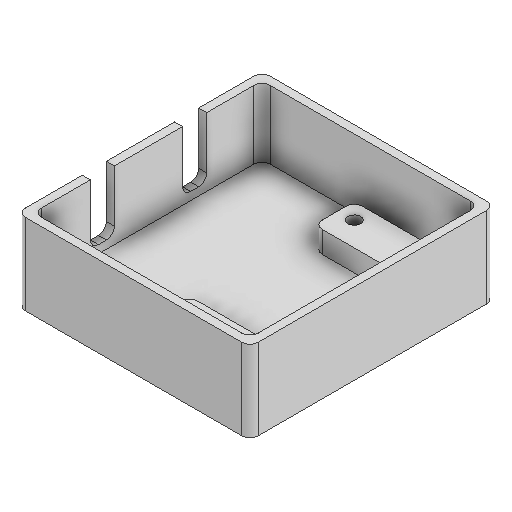
# Autodesk Inventor part: 3DP_ASA_Preamp_Case_Top
Saved by Autodesk Inventor 2026.1 (Build 301233000, 233)
## iProperties
Created: 2025-06-27
Part Number: 3DP_ASA_Preamp_Case_Top
Material: Generic
Document SubType Name: Modeling
Designer: User
Density: 1 g/cm^3
Appearance: Default
Author: User
Autodesk Inventor part; units mm, degrees
ref_plane "YZ Plane" through (0, 0, 0) normal (1, 0, 0) x (0, 1, 0)
ref_plane "XZ Plane" through (0, 0, 0) normal (0, 1, 0) x (-1, 0, 0)
ref_plane "XY Plane" through (0, 0, 0) normal (0, 0, 1) x (1, 0, 0)
sketch "Sketch1" plane through (0, 0, 0) normal (0, 1, 0) x (-1, 0, 0)
  line L0 (12.5, 25.5) -> (-12.5, 25.5)
  line L1 (-12.5, 25.5) -> (-12.5, -25.5)
  line L2 (-12.5, -25.5) -> (12.5, -25.5)
  line L3 (12.5, -25.5) -> (12.5, 25.5)
  line L4 (13, 26) -> (-13, 26)
  line L5 (-13, 26) -> (-13, -26)
  line L6 (-13, -26) -> (13, -26)
  line L7 (13, -26) -> (13, 26)
  line L8 (15, 28) -> (-15, 28)
  line L9 (-15, 28) -> (-15, -28)
  line L10 (-15, -28) -> (15, -28)
  circle A0 centre (8.5, 21.5) radius 1.6
  circle A1 centre (8.5, -21.5) radius 1.6
  circle A2 centre (-8.5, 21.5) radius 1.6
  circle A3 centre (-8.5, -21.5) radius 1.6
  line L11 (15, -28) -> (38, -28)
  line L12 (38, -28) -> (38, -26)
  line L13 (38, -26) -> (13, -26)
  line L14 (13, 26) -> (38, 26)
  line L15 (38, 26) -> (38, 28)
  line L16 (38, 28) -> (15, 28)
  line L17 (38, -26) -> (38, 26)
  line L18 (12.5, -15.5) -> (-12.5, -15.5)
  line L19 (12.5, 15.5) -> (-12.5, 15.5)
  line L20 (12.5, -15.5) -> (13, -15.5)
  line L21 (12.5, 15.5) -> (13, 15.5)
  line L22 (-12.5, -15.5) -> (-13, -15.5)
  line L23 (-12.5, 15.5) -> (-13, 15.5)
  line L24 (38.5, -26) -> (38.5, -28.5)
  line L25 (38.5, -28.5) -> (15, -28.5)
  line L26 (15, -28.5) -> (-15.5, -28.5)
  line L27 (-15.5, -28.5) -> (-15.5, 28.5)
  line L28 (-15.5, 28.5) -> (15, 28.5)
  line L29 (15, 28.5) -> (38.5, 28.5)
  line L30 (38.5, 28.5) -> (38.5, 26)
  line L31 (38.5, -26) -> (38, -26)
  line L32 (38.5, 26) -> (38, 26)
  line L33 (38, 24) -> (40.5, 24)
  line L34 (40.5, 24) -> (40.5, 30.5)
  line L35 (40.5, 30.5) -> (-17.5, 30.5)
  line L36 (-17.5, 30.5) -> (-17.5, -30.5)
  line L37 (-17.5, -30.5) -> (15, -30.5)
  line L38 (15, -30.5) -> (40.5, -30.5)
  line L39 (40.5, -30.5) -> (40.5, -24)
  line L40 (40.5, -24) -> (38, -24)
  line L41 (40.5, -24) -> (40.5, 24)
  line L42 (38.5, -26) -> (38.5, -24)
  line L43 (38.5, -24) -> (38.5, 24)
  line L44 (38.5, 24) -> (38.5, 26)
  point P0 (0, 0)
  dimension "d0" = 51
  dimension "d1" = 25
  dimension "d2" = 12.5
  dimension "d3" = 25.5
  dimension "d4" = 4
  dimension "d5" = 4
  dimension "d6" = 4
  dimension "d7" = 4
  dimension "d8" = 0.5
  dimension "d10" = 3.2
  dimension "d11" = 3.2
  dimension "d12" = 3.2
  dimension "d13" = 3.2
  dimension "d50" = 25
  dimension "d51" = 10
  dimension "d52" = 10
  dimension "d69" = 0.5
  dimension "d70" = 2
  constraints: 90 end point, 18 perpendicular, 11 point on line, 9 parallel, 4 centre point, 4 coincident, 4 horizontal, 2 horizontal alignment, 2 vertical, 2 vertical alignment, 1 collinear, 18 other
  measures "d0" distance between parallel lines of L2 L0
  measures "d1" distance of L1.end L2.end
  measures "d2" distance from line of L3 point (0, 0)
  measures "d3" distance from line of L2 point (0, 0)
  measures "d4" distance from line of L0 point (8.5, 21.5)
  measures "d5" distance from line of L3 point (8.5, 21.5)
  measures "d6" distance from line of L1 point (-8.5, 21.5)
  measures "d7" distance from line of L2 point (8.5, -21.5)
  measures "d8" distance between parallel lines of L3 L7
  measures "d10" diameter of A0
  measures "d11" diameter of A1
  measures "d12" diameter of A2
  measures "d13" diameter of A3
  measures "d50" distance between parallel lines of L17 L7
  measures "d51" distance between parallel lines of L2 L18
  measures "d52" distance between parallel lines of L0 L19
  measures "d69" distance between parallel lines of L11 L25
  measures "d70" distance between parallel lines of L27 L36
extrude "Extrusion1" add sketch "Sketch1" against normal blind 3.2
extrude "Extrusion2" add sketch "Sketch1" along normal blind 17 contours L30 L29 L28 L27 L26 L25 L24 L42 L40 L39 L38 L37 L36 L35 L34 L33 L44 | L33 L41 L40 L43
extrude "Extrusion11" add sketch "Sketch1" along normal blind 5.4 contours L3 L19 L1 L0 | L3 L2 L1 L18
fillet "Fillet6" radius 2 8 edges at (-40.5, 6.9, 30.5) (-40.5, 6.9, -30.5) (17.5, 6.9, -30.5) (17.5, 6.9, 30.5) (15.5, 8.5, 28.5) (15.5, 8.5, -28.5) (-38.5, 8.5, -28.5) (-38.5, 8.5, 28.5)
fillet "Fillet7" radius 2 8 edges at (-12.5, 2.7, -15.5) (-12.5, 2.7, -25.5) (12.5, 2.7, -15.5) (12.5, 2.7, -25.5) (12.5, 2.7, 15.5) (12.5, 2.7, 25.5) (-12.5, 2.7, 25.5) (-12.5, 2.7, 15.5)
sketch "Sketch9" plane through (-40.5, -3.2, -28.5) normal (-1, 0, 0) x (0, 0, 1)
  line L0 (59, 0) -> (59, 20.2) projected
  line L1 (0, 0) -> (0, 20.2) projected
  line L2 (57, 0) -> (0, 0) projected
  line L3 (57, 20.2) -> (57, 0) projected
  line L4 (0, 20.2) -> (57, 20.2) projected
  line L5 (57, 20.2) -> (59, 20.2) projected
  line L6 (59, 0) -> (57, 0) projected
  line L7 (-2, 20.2) -> (0, 20.2) projected
  line L8 (0, 0) -> (-2, 0) projected
  line L9 (-2, 20.2) -> (-2, 0) projected
  line L10 (42.8, 20.2) -> (42.8, 5.2)
  line L11 (42.8, 5.2) -> (36.8, 5.2)
  line L12 (36.8, 5.2) -> (36.8, 20.2)
  line L13 (19.8, 20.2) -> (19.8, 5.2)
  line L14 (19.8, 5.2) -> (13.8, 5.2)
  line L15 (13.8, 5.2) -> (13.8, 20.2)
  point P0 (28.5, 3.2)
  dimension "d75" = 6
  dimension "d76" = 15
  dimension "d77" = 6
  dimension "d78" = 16.2
  dimension "d79" = 17
  constraints: 12 end point, 6 point on line, 3 perpendicular, 1 parallel, 1 vertical
  measures "d75" distance between parallel lines of L12 L10
  measures "d76" distance between parallel lines of L4 L11
  measures "d77" distance between parallel lines of L15 L13
  measures "d78" distance between parallel lines of L10 L0
  measures "d79" distance between parallel lines of L13 L12
extrude "Extrusion12" cut sketch "Sketch9" against normal blind 5.4 contours L10 L11 L12 L4 | L4 L13 L14 L15
fillet "Fillet8" radius 2 4 edges at (-39.5, 2, 14.3) (-39.5, 2, 8.3) (-39.5, 2, -8.7) (-39.5, 2, -14.7)
sketch "Sketch10" plane through (0, -3.2, 0) normal (0, -1, 0) x (1, 0, 0)
  line L0 (-23.4723, 25.4244) -> (-23.4723, -0.8586) construction
  line L1 (-23.4723, -0.8586) -> (-26.6245, -0.8586) construction
  line L2 (-26.6245, -0.8586) -> (-26.6245, 25.4244) construction
  line L3 (-26.6245, 25.4244) -> (-23.4723, 25.4244) construction
  line L4 (-23.5729, 24.8116) -> (-23.5729, 22.4106)
  spline S0 degree 2 poles (-23.5729, 22.4106) (-23.5729, 21.6972) (-23.6918, 20.9975) (-24.0668, 20.4442) (-24.6933, 20.0738) (-25.082, 20.0738) knots 0 0 0 1 2 3 4 4 4
  spline S1 degree 2 poles (-25.082, 20.0738) (-25.5027, 20.0738) (-26.2024, 20.5265) (-26.3808, 20.9152) knots 0 0 0 1 2 2 2
  spline S2 degree 2 poles (-26.3808, 20.9152) (-26.5409, 20.3664) (-27.3091, 19.7811) (-27.8305, 19.7811) knots 0 0 0 1 2 2 2
  spline S3 degree 2 poles (-27.8305, 19.7811) (-28.2421, 19.7811) (-29.0149, 20.1606) (-29.4768, 20.8238) (-29.5317, 21.3039) knots 0 0 0 1 2 3 3 3
  spline S4 degree 2 poles (-29.5317, 21.3039) (-29.5637, 21.6103) (-29.5729, 22.7674) knots 0 0 0 1 1 1
  line L5 (-29.5729, 22.7674) -> (-29.5729, 24.8116)
  line L6 (-29.5729, 24.8116) -> (-23.5729, 24.8116)
  line L7 (-26.9524, 23.5997) -> (-28.5576, 23.5997)
  line L8 (-28.5576, 23.5997) -> (-28.5576, 22.4747)
  spline S5 degree 2 poles (-28.5576, 22.4747) (-28.5576, 21.8161) (-28.521, 21.6424) knots 0 0 0 1 1 1
  spline S6 degree 2 poles (-28.521, 21.6424) (-28.4707, 21.3725) (-28.0912, 21.0295) (-27.771, 21.0295) knots 0 0 0 1 2 2 2
  spline S7 degree 2 poles (-27.771, 21.0295) (-27.5012, 21.0295) (-27.1262, 21.2902) (-26.9524, 21.7887) (-26.9524, 22.6164) knots 0 0 0 1 2 3 3 3
  line L9 (-26.9524, 22.6164) -> (-26.9524, 23.5997)
  line L10 (-24.5698, 23.5997) -> (-25.9555, 23.5997)
  line L11 (-25.9555, 23.5997) -> (-25.9555, 22.8039)
  spline S8 degree 2 poles (-25.9555, 22.8039) (-25.9555, 22.0951) (-25.9372, 21.9213) knots 0 0 0 1 1 1
  spline S9 degree 2 poles (-25.9372, 21.9213) (-25.896, 21.6103) (-25.5439, 21.2536) (-25.2512, 21.2536) knots 0 0 0 1 2 2 2
  spline S10 degree 2 poles (-25.2512, 21.2536) (-24.9723, 21.2536) (-24.6293, 21.56) (-24.5881, 21.8664) knots 0 0 0 1 2 2 2
  spline S11 degree 2 poles (-24.5881, 21.8664) (-24.5698, 22.0448) (-24.5698, 22.9045) knots 0 0 0 1 1 1
  line L12 (-24.5698, 22.9045) -> (-24.5698, 23.5997)
  line L13 (-29.5729, 17.1835) -> (-27.0485, 17.1835)
  line L14 (-27.0485, 17.1835) -> (-23.5729, 19.3786)
  line L15 (-23.5729, 19.3786) -> (-23.5729, 17.9609)
  line L16 (-23.5729, 17.9609) -> (-25.9509, 16.5433)
  line L17 (-25.9509, 16.5433) -> (-23.5729, 15.1622)
  line L18 (-23.5729, 15.1622) -> (-23.5729, 13.7628)
  line L19 (-23.5729, 13.7628) -> (-27.0576, 15.9716)
  line L20 (-27.0576, 15.9716) -> (-29.5729, 15.9716)
  line L21 (-29.5729, 15.9716) -> (-29.5729, 17.1835)
  line L22 (-29.5729, 11.8146) -> (-24.5881, 11.8146)
  line L23 (-24.5881, 11.8146) -> (-24.5881, 13.5936)
  line L24 (-24.5881, 13.5936) -> (-23.5729, 13.5936)
  line L25 (-23.5729, 13.5936) -> (-23.5729, 8.8283)
  line L26 (-23.5729, 8.8283) -> (-24.5881, 8.8283)
  line L27 (-24.5881, 8.8283) -> (-24.5881, 10.6027)
  line L28 (-24.5881, 10.6027) -> (-29.5729, 10.6027)
  line L29 (-29.5729, 10.6027) -> (-29.5729, 11.8146)
  line L30 (-29.5729, 8.0417) -> (-23.5729, 8.0417)
  line L31 (-23.5729, 8.0417) -> (-23.5729, 3.592)
  line L32 (-23.5729, 3.592) -> (-24.5881, 3.592)
  line L33 (-24.5881, 3.592) -> (-24.5881, 6.8299)
  line L34 (-24.5881, 6.8299) -> (-25.9189, 6.8299)
  line L35 (-25.9189, 6.8299) -> (-25.9189, 3.8161)
  line L36 (-25.9189, 3.8161) -> (-26.9341, 3.8161)
  line L37 (-26.9341, 3.8161) -> (-26.9341, 6.8299)
  line L38 (-26.9341, 6.8299) -> (-28.5576, 6.8299)
  line L39 (-28.5576, 6.8299) -> (-28.5576, 3.4777)
  line L40 (-28.5576, 3.4777) -> (-29.5729, 3.4777)
  line L41 (-29.5729, 3.4777) -> (-29.5729, 8.0417)
  line L42 (-27.364, -1.3881) -> (-27.7345, -2.5634)
  spline S12 degree 2 poles (-27.7345, -2.5634) (-28.7177, -2.2936) (-29.6735, -1.036) (-29.6735, -0.0711) knots 0 0 0 1 2 2 2
  spline S13 degree 2 poles (-29.6735, -0.0711) (-29.6735, 1.1225) (-28.0409, 2.6637) (-26.6277, 2.6637) knots 0 0 0 1 2 2 2
  spline S14 degree 2 poles (-26.6277, 2.6637) (-25.1277, 2.6637) (-23.4723, 1.118) (-23.4723, -0.1442) knots 0 0 0 1 2 2 2
  spline S15 degree 2 poles (-23.4723, -0.1442) (-23.4723, -1.2418) (-24.1216, -1.9323) knots 0 0 0 1 1 1
  spline S16 degree 2 poles (-24.1216, -1.9323) (-24.5058, -2.3394) (-25.2238, -2.5451) knots 0 0 0 1 1 1
  line L43 (-25.2238, -2.5451) -> (-25.5119, -1.347)
  spline S17 degree 2 poles (-25.5119, -1.347) (-25.0454, -1.2418) (-24.5058, -0.565) (-24.5058, -0.0848) knots 0 0 0 1 2 2 2
  spline S18 degree 2 poles (-24.5058, -0.0848) (-24.5058, 0.5829) (-25.4616, 1.4152) (-26.5363, 1.4152) knots 0 0 0 1 2 2 2
  spline S19 degree 2 poles (-26.5363, 1.4152) (-27.675, 1.4152) (-28.6399, 0.5966) (-28.6399, -0.0573) knots 0 0 0 1 2 2 2
  spline S20 degree 2 poles (-28.6399, -0.0573) (-28.6399, -0.5421) (-28.0226, -1.2372) (-27.364, -1.3881) knots 0 0 0 1 2 2 2
  line L44 (-29.5729, -3.6061) -> (-23.5729, -3.6061)
  line L45 (-23.5729, -3.6061) -> (-23.5729, -4.818)
  line L46 (-23.5729, -4.818) -> (-25.9326, -4.818)
  line L47 (-25.9326, -4.818) -> (-25.9326, -7.1915)
  line L48 (-25.9326, -7.1915) -> (-23.5729, -7.1915)
  line L49 (-23.5729, -7.1915) -> (-23.5729, -8.4034)
  line L50 (-23.5729, -8.4034) -> (-29.5729, -8.4034)
  line L51 (-29.5729, -8.4034) -> (-29.5729, -7.1915)
  line L52 (-29.5729, -7.1915) -> (-26.9479, -7.1915)
  line L53 (-26.9479, -7.1915) -> (-26.9479, -4.818)
  line L54 (-26.9479, -4.818) -> (-29.5729, -4.818)
  line L55 (-29.5729, -4.818) -> (-29.5729, -3.6061)
  line L56 (-29.5729, -9.693) -> (-23.6232, -9.693)
  line L57 (-23.6232, -9.693) -> (-23.6232, -10.9049)
  line L58 (-23.6232, -10.9049) -> (-28.5576, -10.9049)
  line L59 (-28.5576, -10.9049) -> (-28.5576, -13.9186)
  line L60 (-28.5576, -13.9186) -> (-29.5729, -13.9186)
  line L61 (-29.5729, -13.9186) -> (-29.5729, -9.693)
  line L62 (-29.5729, -20.1884) -> (-29.5729, -18.8714)
  line L63 (-29.5729, -18.8714) -> (-28.2101, -18.35)
  line L64 (-28.2101, -18.35) -> (-28.2101, -15.9537)
  line L65 (-28.2101, -15.9537) -> (-29.5729, -15.4552)
  line L66 (-29.5729, -15.4552) -> (-29.5729, -14.1702)
  line L67 (-29.5729, -14.1702) -> (-23.5729, -16.5025)
  line L68 (-23.5729, -16.5025) -> (-23.5729, -17.7921)
  line L69 (-23.5729, -17.7921) -> (-29.5729, -20.1884)
  line L70 (-27.1948, -17.9613) -> (-24.9723, -17.1336)
  line L71 (-24.9723, -17.1336) -> (-27.1948, -16.3195)
  line L72 (-27.1948, -16.3195) -> (-27.1948, -17.9613)
  line L73 (-23.5729, -20.8378) -> (-23.5729, -23.2387)
  spline S21 degree 2 poles (-23.5729, -23.2387) (-23.5729, -23.9522) (-23.6918, -24.6519) (-24.0668, -25.2052) (-24.6933, -25.5756) (-25.082, -25.5756) knots 0 0 0 1 2 3 4 4 4
  spline S22 degree 2 poles (-25.082, -25.5756) (-25.5027, -25.5756) (-26.2024, -25.1229) (-26.3808, -24.7342) knots 0 0 0 1 2 2 2
  spline S23 degree 2 poles (-26.3808, -24.7342) (-26.5409, -25.283) (-27.3091, -25.8683) (-27.8305, -25.8683) knots 0 0 0 1 2 2 2
  spline S24 degree 2 poles (-27.8305, -25.8683) (-28.2421, -25.8683) (-29.0149, -25.4887) (-29.4768, -24.8256) (-29.5317, -24.3455) knots 0 0 0 1 2 3 3 3
  spline S25 degree 2 poles (-29.5317, -24.3455) (-29.5637, -24.0391) (-29.5729, -22.882) knots 0 0 0 1 1 1
  line L74 (-29.5729, -22.882) -> (-29.5729, -20.8378)
  line L75 (-29.5729, -20.8378) -> (-23.5729, -20.8378)
  line L76 (-26.9524, -22.0497) -> (-28.5576, -22.0497)
  line L77 (-28.5576, -22.0497) -> (-28.5576, -23.1747)
  spline S26 degree 2 poles (-28.5576, -23.1747) (-28.5576, -23.8333) (-28.521, -24.007) knots 0 0 0 1 1 1
  spline S27 degree 2 poles (-28.521, -24.007) (-28.4707, -24.2769) (-28.0912, -24.6198) (-27.771, -24.6198) knots 0 0 0 1 2 2 2
  spline S28 degree 2 poles (-27.771, -24.6198) (-27.5012, -24.6198) (-27.1262, -24.3592) (-26.9524, -23.8607) (-26.9524, -23.033) knots 0 0 0 1 2 3 3 3
  line L78 (-26.9524, -23.033) -> (-26.9524, -22.0497)
  line L79 (-24.5698, -22.0497) -> (-25.9555, -22.0497)
  line L80 (-25.9555, -22.0497) -> (-25.9555, -22.8455)
  spline S29 degree 2 poles (-25.9555, -22.8455) (-25.9555, -23.5543) (-25.9372, -23.7281) knots 0 0 0 1 1 1
  spline S30 degree 2 poles (-25.9372, -23.7281) (-25.896, -24.0391) (-25.5439, -24.3958) (-25.2512, -24.3958) knots 0 0 0 1 2 2 2
  spline S31 degree 2 poles (-25.2512, -24.3958) (-24.9723, -24.3958) (-24.6293, -24.0894) (-24.5881, -23.783) knots 0 0 0 1 2 2 2
  spline S32 degree 2 poles (-24.5881, -23.783) (-24.5698, -23.6046) (-24.5698, -22.7448) knots 0 0 0 1 1 1
  line L81 (-24.5698, -22.7448) -> (-24.5698, -22.0497)
  point P0 (0, 0)
  constraints: 2 other
extrude "Extrusion13" cut sketch "Sketch10" against normal blind 0.2
equation "\"d2\" = 0.5 * d1"
equation "\"d3\" = 0.5 * d0"
equation "\"d5\" = d4"
equation "\"d6\" = d5"
equation "\"d7\" = d4"
equation "\"d10\" = d12"
equation "\"d11\" = d12"
equation "\"d13\" = d12"
equation "\"d14\" = d12"
equation "\"d77\" = d75"
body "Solid1"
